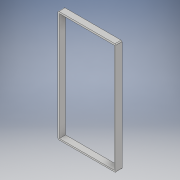
# Autodesk Inventor part: Smart Lock Box Middle Correct
Saved by Autodesk Inventor 2019.3 (Build 233278000, 278)
## iProperties
Created: 2019-04-11
Part Number: Smart Lock Box Middle Correct
Material: Generic
Document SubType Name: Modeling
Designer: grego
Density: 1 g/cm^3
Appearance: Default
Author: grego
Autodesk Inventor part; units mm, degrees
ref_plane "YZ Plane" through (0, 0, 0) normal (1, 0, 0) x (0, 1, 0)
ref_plane "XZ Plane" through (0, 0, 0) normal (0, 1, 0) x (-1, 0, 0)
ref_plane "XY Plane" through (0, 0, 0) normal (0, 0, 1) x (1, 0, 0)
sketch "Sketch1" plane through (0, 0, 0) normal (0, 0, 1) x (1, 0, 0)
  line L0 (-66.6872, 56.6432) -> (-66.6872, -62.4828)
  line L1 (-66.6872, -62.4828) -> (-4.7112, -62.4828)
  line L2 (-4.7112, -62.4828) -> (-4.7112, 56.6432)
  line L3 (-4.7112, 56.6432) -> (-66.6872, 56.6432)
  point P0 (0, 0)
  dimension "d0" = 119.126
  dimension "d1" = 61.976
  constraints: 8 end point, 3 perpendicular, 1 vertical
  measures "d0" distance between parallel lines of L1 L3
  measures "d1" distance between parallel lines of L2 L0
extrude "Extrusion1" add sketch "Sketch1" along normal blind 6.604
sketch "Sketch2" plane through (0, 0, 6.604) normal (0, 0, 1) x (1, 0, 0)
  line L0 (-65.1652, 54.8612) -> (-6.2352, 54.8612)
  line L1 (-6.2352, 54.8612) -> (-6.2352, -60.9588)
  line L2 (-6.2352, -60.9588) -> (-65.1652, -60.9588)
  line L3 (-65.1652, -60.9588) -> (-65.1652, 54.8612)
  line L4 (-4.7112, -62.4828) -> (-4.7112, 56.6432) projected
  line L5 (-66.6872, -62.4828) -> (-4.7112, -62.4828) projected
  point P0 (0, 0)
  dimension "d4" = 115.82
  dimension "d5" = 58.93
  dimension "d6" = 1.524
  dimension "d7" = 1.524
  constraints: 8 end point, 2 parallel, 1 horizontal, 1 perpendicular
  measures "d4" distance between parallel lines of L2 L0
  measures "d5" distance between parallel lines of L3 L1
  measures "d6" distance between parallel lines of L4 L1
  measures "d7" distance between parallel lines of L5 L2
extrude "Extrusion2" cut sketch "Sketch2" against normal blind 6.604
fillet "Fillet1" radius 1 4 edges at (-66.6872, -62.4828, 3.302) (-66.6872, 56.6432, 3.302) (-4.7112, 56.6432, 3.302) (-4.7112, -62.4828, 3.302)
body "Solid1"
